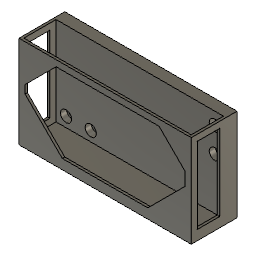
USB分割ハブホルダー 壁型 v1 (Autodesk Fusion 360 design; units mm, degrees)
Autodesk Fusion 360 part; units mm, degrees
sketch "スケッチ1" plane through (0, 0, 0) normal (0, 0, 1) x (1, 0, 0)
  line L0 (0, 0) -> (2, 0)
  line L1 (2, 0) -> (137, 0)
  line L2 (137, 0) -> (137, 2)
  line L3 (137, 2) -> (2, 2)
  line L4 (2, 2) -> (2, 0)
  line L5 (2, 0) -> (0, 0)
  line L6 (0, 0) -> (0, 28)
  line L7 (0, 28) -> (2, 28)
  line L8 (2, 28) -> (2, 0)
  line L9 (137, 0) -> (139, 0)
  line L10 (139, 0) -> (139, 28)
  line L11 (139, 28) -> (137, 28)
  line L12 (137, 28) -> (137, 0)
  line L13 (139, 0) -> (134, 0)
  line L14 (134, 0) -> (134, 5)
  line L15 (134, 5) -> (139, 5)
  line L16 (139, 5) -> (139, 0)
  line L17 (0, 0) -> (5, 0)
  line L18 (5, 0) -> (5, 5)
  line L19 (5, 5) -> (0, 5)
  line L20 (0, 5) -> (0, 0)
  line L21 (0, 28) -> (2, 28)
  line L22 (2, 28) -> (2, 23)
  line L23 (2, 23) -> (0, 23)
  line L24 (0, 23) -> (0, 28)
  line L25 (137, 28) -> (139, 28)
  line L26 (139, 28) -> (139, 23)
  line L27 (139, 23) -> (137, 23)
  line L28 (137, 23) -> (137, 28)
  line L29 (0, 28) -> (139, 28)
  line L30 (139, 28) -> (139, 0)
  line L31 (139, 0) -> (0, 0)
  line L32 (0, 0) -> (0, 28)
  dimension "d12" = 2
  dimension "d14" = 135
  dimension "d15" = 2
  dimension "d16" = 28
  dimension "d17" = 2
  dimension "d18" = 28
  dimension "d19" = 5
  dimension "d20" = 5
  dimension "d21" = 5
  dimension "d22" = 5
  dimension "d23" = 2
  dimension "d24" = 5
  dimension "d25" = 2
  dimension "d26" = 5
  constraint horizontal L0
  constraint coincident L0.start L5.end
  constraint horizontal L1
  constraint vertical L2
  constraint horizontal L3
  constraint vertical L4
  constraint horizontal L5
  constraint vertical L6
  constraint horizontal L7
  constraint vertical L8
  constraint horizontal L9
  constraint vertical L10
  constraint horizontal L11
  constraint vertical L12
  constraint horizontal L13
  constraint vertical L14
  constraint horizontal L15
  constraint vertical L16
  constraint horizontal L17
  constraint vertical L18
  constraint horizontal L19
  constraint vertical L20
  constraint horizontal L21
  constraint vertical L22
  constraint horizontal L23
  constraint vertical L24
  constraint horizontal L25
  constraint vertical L26
  constraint horizontal L27
  constraint vertical L28
  constraint horizontal L29
  constraint vertical L30
  constraint horizontal L31
  constraint vertical L32
  measures "d12" distance of L0.start L0.end
  measures "d14" distance of L0.end L1.end
  measures "d15" distance of L0.end L3.end
  measures "d16" distance of L0.end L7.end
  measures "d17" distance of L1.end L9.end
  measures "d18" distance of L1.end L11.end
  measures "d19" distance of L9.end L13.end
  measures "d20" distance of L9.end L15.end
  measures "d21" distance of L0.start L17.end
  measures "d22" distance of L0.start L19.end
  measures "d23" distance of L6.end L7.end
  measures "d24" distance of L6.end L23.end
  measures "d25" distance of L11.end L10.end
  measures "d26" distance of L11.end L27.end
extrude "押し出し4" add sketch "スケッチ1" along normal blind 5 contours L6 L8 L19 L23 L32 | L1 L3 L14 L18 L31 | L10 L12 L15 L27 L30 makes body 1 at (0, 11, 1.6667) makes body 2 at (91, 2, 1.6667) makes body 3 at (137, 17, 1.6667)
extrude "押し出し5" add sketch "スケッチ1" along normal blind 71.5 contours L0 L4 L5 L6 L8 L17 L19 L20 L31 L32 | L1 L3 L4 L8 L17 L18 L31 | L6 L7 L8 L21 L22 L23 L24 L29 L32 | L1 L2 L3 L12 L13 L14 L31 | L2 L9 L10 L12 L13 L15 L16 L30 L31 | L10 L11 L12 L25 L26 L27 L28 L29 L30 bodies 1 2 3
extrude "押し出し6" add sketch "スケッチ1" against normal blind 3 bodies 1
sketch "スケッチ2" plane through (139, 0, 0) normal (1, 0, 0) x (0, 1, 0)
  line L0 (28, -3) -> (28, 71.5)
  line L1 (28, 71.5) -> (23, 71.5)
  line L2 (23, 71.5) -> (23, 5)
  line L3 (23, 5) -> (5, 5)
  line L4 (5, 5) -> (5, 71.5)
  line L5 (5, 71.5) -> (0, 71.5)
  line L6 (0, 71.5) -> (0, -3)
  line L7 (0, -3) -> (28, -3)
  line L8 (5, 5) -> (5, 35)
  line L9 (5, 35) -> (35, 5)
  line L10 (23, 5) -> (23, -7.9001)
  line L11 (23, -7.9001) -> (28.8124, 5)
  line L12 (5, 71.5) -> (5, 64.5296)
  line L13 (5, 71.5) -> (95.3571, 71.5)
  line L14 (95.3571, 71.5) -> (95.3571, 66.5)
  line L15 (95.3571, 66.5) -> (5, 66.5)
  line L16 (5, 66.5) -> (5, 71.5)
  line L17 (5, 64.5296) -> (11.561, 66.5)
  line L18 (23, 71.5) -> (23, 103.8563)
  line L19 (23, 103.8563) -> (38.5847, 66.5)
  dimension "d78" = 5
  constraint coincident L3.end L4.start
  constraint coincident L4 L8.end
  constraint perpendicular L3 L8
  constraint coincident L3 L9.end
  constraint coincident L2.end L3.start
  constraint coincident L2 L10.end
  constraint perpendicular L3 L10
  constraint coincident L3 L11.end
  constraint coincident L4.end L5.start
  constraint perpendicular L5 L12
  constraint horizontal L13
  constraint vertical L14
  constraint horizontal L15
  constraint vertical L16
  constraint coincident L15 L17.end
  constraint coincident L1.end L2.start
  constraint perpendicular L13 L18
  constraint coincident L15 L19.end
  measures "d78" distance of L4.end L15.end
sketch "スケッチ3" plane through (0, 0, 0) normal (-1, 0, 0) x (0, -1, 0)
  line L0 (0, -3) -> (0, 71.5)
  line L1 (0, 71.5) -> (-5, 71.5)
  line L2 (-5, 71.5) -> (-5, 5)
  line L3 (-5, 5) -> (-23, 5)
  line L4 (-23, 5) -> (-23, 71.5)
  line L5 (-23, 71.5) -> (-28, 71.5)
  line L6 (-28, 71.5) -> (-28, -3)
  line L7 (-28, -3) -> (0, -3)
  line L8 (-23, 5) -> (-23, -7.9001)
  line L9 (-23, -7.9001) -> (-28.8124, 5)
  line L10 (-5, 5) -> (-5, 35)
  line L11 (-5, 35) -> (-35, 5)
  line L12 (-23, 71.5) -> (-23, 36.5)
  line L13 (-23, 71.5) -> (8.1643, 71.5)
  line L14 (8.1643, 71.5) -> (8.1643, 66.5)
  line L15 (8.1643, 66.5) -> (-23, 66.5)
  line L16 (-23, 66.5) -> (-23, 71.5)
  line L17 (-23, 36.5) -> (-73.5896, 66.5)
  line L18 (8.1643, 66.5) -> (8.1643, 36.5)
  line L19 (8.1643, 36.5) -> (-43.3484, 66.5)
  line L20 (8.1643, 36.5) -> (37.4264, 36.5) construction
  dimension "d83" = 35
  dimension "d84" = 5
  dimension "d86" = 30
  constraint coincident L3.end L4.start
  constraint coincident L4 L8.end
  constraint perpendicular L3 L8
  constraint coincident L3 L9.end
  constraint coincident L2.end L3.start
  constraint coincident L2 L10.end
  constraint perpendicular L3 L10
  constraint coincident L3 L11.end
  constraint coincident L4.end L5.start
  constraint coincident L4 L12.end
  constraint horizontal L13
  constraint vertical L14
  constraint horizontal L15
  constraint vertical L16
  constraint coincident L15 L17.end
  constraint perpendicular L15 L18
  constraint horizontal L20
  constraint coincident L15 L19.end
  measures "d83" distance of L4.end L12.end
  measures "d84" distance of L4.end L15.end
  measures "d86" distance of L14.end L18.end
sketch "スケッチ4" plane through (0, 0, 0) normal (0, -1, 0) x (1, 0, 0)
  line L0 (139, -3) -> (139, 71.5)
  line L1 (139, 71.5) -> (134, 71.5)
  line L2 (134, 71.5) -> (134, 5)
  line L3 (134, 5) -> (5, 5)
  line L4 (5, 5) -> (5, 71.5)
  line L5 (5, 71.5) -> (0, 71.5)
  line L6 (0, 71.5) -> (0, -3)
  line L7 (0, -3) -> (139, -3)
  line L8 (5, 5) -> (5, 35)
  line L9 (5, 35) -> (35, 5)
  line L10 (134, 5) -> (134, 35)
  line L11 (134, 35) -> (104, 5)
  line L12 (5, 71.5) -> (138.0686, 71.5)
  line L13 (138.0686, 71.5) -> (138.0686, 66.5)
  line L14 (138.0686, 66.5) -> (5, 66.5)
  line L15 (5, 66.5) -> (5, 71.5)
  line L16 (5, 66.5) -> (5, 41.5)
  line L17 (5, 41.5) -> (30, 66.5)
  line L18 (5, 41.5) -> (40.3553, 41.5) construction
  line L19 (138.0686, 66.5) -> (138.0686, 41.5)
  line L20 (138.0686, 41.5) -> (113.0686, 66.5)
  line L21 (138.0686, 41.5) -> (167.8553, 41.5) construction
  dimension "d33" = 45
  dimension "d39" = 5
  dimension "d40" = 25
  dimension "d41" = 45
  dimension "d42" = 25
  dimension "d43" = 135
  constraint coincident L3.end L4.start
  constraint coincident L4 L8.end
  constraint perpendicular L3 L8
  constraint coincident L3 L9.end
  constraint coincident L2.end L3.start
  constraint coincident L2 L10.end
  constraint perpendicular L3 L10
  constraint coincident L3 L11.end
  constraint horizontal L12
  constraint vertical L13
  constraint horizontal L14
  constraint vertical L15
  constraint coincident L4.end L5.start
  constraint perpendicular L14 L16
  constraint horizontal L18
  constraint coincident L14 L17.end
  constraint perpendicular L14 L19
  constraint horizontal L21
  constraint coincident L14 L20.end
  measures "d33" angle of L10 L11
  measures "d39" distance of L4.end L14.end
  measures "d40" distance of L14.end L16.end
  measures "d41" angle of L17 L18
  measures "d42" distance of L13.end L19.end
  measures "d43" angle of L20 L21
extrude "押し出し7" add sketch "スケッチ2" against normal blind 2 contours L0 L7 L11 | L0 L2 L7 L9 L10 L11 | L0 L2 L9 L15 | L3 L4 L5 L6 L7 L8 L10 L12 L16 | L0 L1 L2 L13 L15 | L2 L4 L12 L13 L15 L16 bodies 1
extrude "押し出し8" add sketch "スケッチ3" against normal blind 2 contours L0 L2 L3 L7 L8 L10 L19 | L0 L2 L15 L19 | L4 L6 L7 L8 L9 L11 | L0 L1 L2 L13 L15 | L6 L7 L9 | L2 L4 L12 L13 L15 L16 | L4 L5 L6 L12 L16 L19 | L4 L6 L12 L17 L19 | L4 L6 L11 L17 bodies 1
extrude "押し出し9" add sketch "スケッチ4" against normal blind 2 contours L2 L4 L12 L14 L15 | L2 L14 L20 | L4 L14 L16 L17 | L2 L3 L10 L11 | L3 L4 L8 L9 bodies 1
sketch "スケッチ5" plane through (0, 28, 0) normal (0, 1, 0) x (-1, 0, 0)
  line L0 (-137, 0) -> (-137, 71.5)
  line L1 (-137, 71.5) -> (-139, 71.5)
  line L2 (-139, 71.5) -> (-139, -3)
  line L3 (-139, -3) -> (0, -3)
  line L4 (0, -3) -> (0, 71.5)
  line L5 (-2, 71.5) -> (-2, 0)
  line L6 (-2, 0) -> (-137, 0)
  line L7 (-40, 15) -> (-40, -43)
  line L8 (-40, -43) -> (0, -43)
  line L9 (0, -43) -> (0, -3)
  line L10 (-13, 15) -> (-13, -43)
  line L11 (-13, -43) -> (-7, -43)
  line L12 (-7, -43) -> (-7, 15)
  line L13 (-33, 15) -> (-27, 15)
  line L14 (-27, 15) -> (-27, -43)
  line L15 (-27, -43) -> (-33, -43)
  line L16 (-33, -43) -> (-33, 15)
  line L17 (-27, 15) -> (-13, 15)
  line L18 (-40, 15) -> (0, 15)
  line L19 (0, 15) -> (0, 0)
  line L20 (0, 0) -> (-40, 0)
  line L21 (-40, 0) -> (-40, 15)
  circle A0 centre (-30, 8) radius 2.8
  circle A1 centre (-10, 8) radius 2.8
  line L22 (-139, 71.5) -> (-179, 71.5)
  line L23 (-179, 71.5) -> (-179, 31.5)
  line L24 (-179, 31.5) -> (-139, 31.5)
  line L25 (-139, 31.5) -> (-139, 71.5)
  line L26 (-139, 71.5) -> (-139, 61.5)
  line L27 (-139, 31.5) -> (-139, 41.5)
  line L28 (-30, 15) -> (-30, 8)
  line L29 (-139, 71.5) -> (-154, 71.5)
  line L30 (-154, 71.5) -> (-154, 31.5)
  line L31 (-139, 61.5) -> (-130, 61.5)
  line L32 (-139, 41.5) -> (-130, 41.5)
  circle A2 centre (-130, 61.5) radius 2.8
  circle A3 centre (-130, 41.5) radius 2.8
  line L33 (-139, 71.5) -> (-122, 71.5)
  line L34 (-122, 71.5) -> (-122, 92.8768)
  line L35 (-122, 92.8768) -> (-139, 92.8768)
  line L36 (-139, 92.8768) -> (-139, 71.5)
  line L37 (0, -3) -> (-139, -3)
  line L38 (-139, -3) -> (-139, 71.5)
  line L39 (-139, 71.5) -> (0, 71.5)
  line L40 (0, 71.5) -> (0, -3)
  line L41 (0, 71.5) -> (-2, 71.5)
  dimension "d47" = 40
  dimension "d50" = 6
  dimension "d51" = 6
  dimension "d52" = 5.6
  dimension "d53" = 5.6
  dimension "d54" = 40
  dimension "d55" = 40
  dimension "d56" = 10
  dimension "d57" = 10
  dimension "d62" = 15
  dimension "d69" = 9
  dimension "d70" = 9
  dimension "d71" = 5.6
  dimension "d72" = 5.6
  dimension "d73" = 17
  constraint vertical L7
  constraint horizontal L8
  constraint vertical L9
  constraint coincident L3.end L4.start
  constraint vertical L10
  constraint horizontal L11
  constraint vertical L12
  constraint horizontal L13
  constraint vertical L14
  constraint horizontal L15
  constraint vertical L16
  constraint perpendicular L10 L17
  constraint horizontal L18
  constraint vertical L19
  constraint horizontal L20
  constraint vertical L21
  constraint coincident L9 L19.end
  constraint horizontal L22
  constraint vertical L23
  constraint horizontal L24
  constraint vertical L25
  constraint coincident L1.end L2.start
  constraint perpendicular L1 L26
  constraint perpendicular L24 L27
  constraint midpoint L13 L28.start
  constraint coincident A0.centre L28.end
  constraint perpendicular L25 L29
  constraint coincident L24 L30.end
  constraint perpendicular L24 L30
  constraint perpendicular L0 L31
  constraint perpendicular L27 L32
  constraint coincident L31.end A2.centre
  constraint coincident L32.end A3.centre
  constraint horizontal L33
  constraint vertical L34
  constraint horizontal L35
  constraint vertical L36
  constraint horizontal L37
  constraint vertical L38
  constraint horizontal L39
  constraint vertical L40
  measures "d47" distance of L3.end L8.end
  measures "d50" distance of L12.end L10.start
  measures "d51" distance of L13.start L13.end
  measures "d52" diameter of A0
  measures "d53" diameter of A1
  measures "d54" distance of L1.end L22.end
  measures "d55" distance of L1.end L24.end
  measures "d56" distance of L1.end L26.end
  measures "d57" distance of L24.end L27.end
  measures "d62" distance of L1.end L29.end
  measures "d69" distance of L26.end L31.end
  measures "d70" distance of L27.end L32.end
  measures "d71" diameter of A2
  measures "d72" diameter of A3
  measures "d73" distance of L1.end L33.end
extrude "押し出し11" add sketch "スケッチ5" along normal blind 9 contours L0 L2 L3 L6 L7 L25 L27 L32 L37 L38 | L0 L5 L6 L7 L13 L17 L18 L21 L33 L39 | L0 L2 L25 L31 L32 L38 | L6 L7 L16 L18 L20 L21 | L3 L6 L7 L16 L20 L37 | L0 L1 L2 L25 L26 L31 L33 L38 L39 | L6 L13 L14 L16 L18 L20 | L3 L6 L14 L16 L20 L37 | L6 L10 L14 L17 L18 L20 | L3 L6 L10 L14 L20 L37 | L6 L10 L12 L18 L20 | L3 L6 L10 L12 L20 L37 | L4 L5 L18 L39 L40 L41 | L5 L6 L12 L18 L20 | L3 L4 L6 L12 L20 L37 L40 | L4 L5 L18 L19 L20 L40 bodies 1
sketch "スケッチ6" plane through (0, 28, 0) normal (0, -1, 0) x (1, 0, 0)
  line L0 (2, 71.5) -> (2, 0)
  line L1 (2, 0) -> (137, 0)
  line L2 (137, 0) -> (137, 71.5)
  line L3 (137, 71.5) -> (2, 71.5)
  circle A0 centre (30, 8) radius 2.8
  circle A1 centre (10, 8) radius 2.8
  circle A2 centre (130, 41.5) radius 2.8
  circle A3 centre (130, 61.5) radius 2.8
  circle A4 centre (30, 8) radius 4.5
  circle A5 centre (10, 8) radius 4.5
  circle A6 centre (130, 61.5) radius 4.5
  circle A7 centre (130, 41.5) radius 4.5
  dimension "d88" = 9
  dimension "d89" = 9
  dimension "d90" = 9
  dimension "d91" = 9
  constraint concentric A0 A4
  constraint concentric A1 A5
  constraint concentric A3 A6
  constraint concentric A2 A7
  measures "d88" diameter of A4
  measures "d89" diameter of A5
  measures "d90" diameter of A6
  measures "d91" diameter of A7
extrude "押し出し12" cut sketch "スケッチ6" against normal blind 5 contours A4 | A5 | A6 | A7 bodies 1
move_body "移動1" [no effect]
